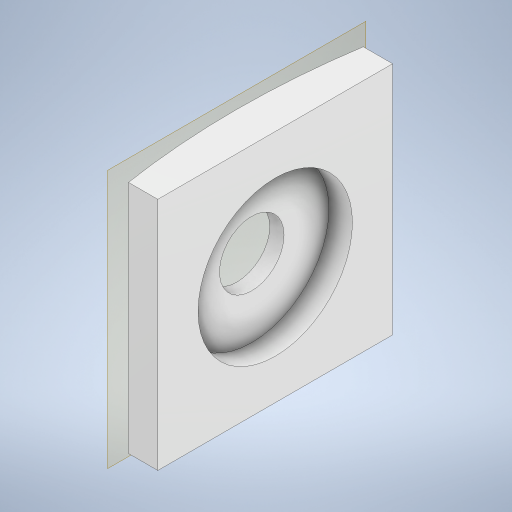
# Autodesk Inventor part: shift_fixed_socket
Saved by Autodesk Inventor 2023 (Build 270158000, 158)
## iProperties
Created: 2023-07-22
Part Number: shift_fixed_socket
Material: Acetal Resin, White
Document SubType Name: Modeling
Designer: 310611102
Density: 1.425 g/cm^3
Appearance: Smooth - White
Mass: 10.3879 g
Surface Area: 43.1103 cm^2
Volume: 7.28974 cm^3
Author: 310611102
Autodesk Inventor part; units mm, degrees
ref_plane "XZ Plane" through (0, 0, 0) normal (0, 1, 0) x (-1, 0, 0)
ref_plane "XY Plane" through (0, 0, 0) normal (0, 0, 1) x (1, 0, 0)
sketch "Sketch1" plane through (0, 0, 0) normal (0, 1, 0) x (-1, 0, 0)
  arc A0 (128.4523, -20) -> (128.4523, 20) centre (0, 0) ccw
  line L0 (128.4523, 20) -> (123.4523, 20)
  line L1 (123.4523, 20) -> (123.4523, -20)
  line L2 (123.4523, -20) -> (128.4523, -20)
  point P0 (123.4523, 0)
  dimension "d0" = 130
  dimension "d1" = 40
  dimension "d2" = 5
  constraints: 6 end point, 2 perpendicular, 2 point on circle, 1 centre point, 1 coincident, 1 horizontal, 1 horizontal alignment, 1 midpoint
  measures "d0" radius of A0
  measures "d1" distance of L0.end L1.end
  measures "d2" distance of L1.end L2.end
extrude "Extrusion1" add sketch "Sketch1" along normal blind 40
sketch "Sketch2" plane through (-123.4523, 0, 20) normal (1, 0, 0) x (0, 0, -1)
  circle A0 centre (20, 20) radius 13.15
  line L0 (0, 0) -> (0, 40) projected
  line L1 (0, 0) -> (40, 0) projected
  point P0 (20, 0)
  point P1 (0, 20)
  point P2 (20, 0)
  dimension "d5" = 26.3
  constraints: 2 midpoint, 1 centre point, 1 horizontal alignment, 1 vertical alignment
  measures "d5" diameter of A0
extrude "Extrusion2" cut sketch "Sketch2" against normal blind 4
sketch "Sketch3" plane through (-127.4523, 20, 0) normal (1, 0, 0) x (0, 0, -1)
  circle A0 centre (0, 0) radius 5.5
  point P0 (0, -20)
  dimension "d8" = 11
  constraints: 1 centre point
  measures "d8" diameter of A0
extrude "Extrusion3" cut sketch "Sketch3" against normal through all
ref_plane "Work Plane1" through (-130, 0, 0) normal (1, 0, 0) x (0, 1, 0)
sketch "Sketch4" plane through (-130, 0, 0) normal (1, 0, 0) x (0, 1, 0)
  circle A0 centre (34.1421, -14.1421) radius 1.5
  circle A1 centre (20, 0) radius 5.5 projected
  circle A2 centre (20, 0) radius 20 construction
  circle A3 centre (34.1421, 14.1421) radius 1.5
  circle A4 centre (5.8579, 14.1421) radius 1.5
  circle A5 centre (5.8579, -14.1421) radius 1.5
  line L0 (20, 0) -> (20, -24.623) construction
  line L1 (20, 0) -> (34.1421, -14.1421) construction
  point P0 (0, 0)
  dimension "d15" = 40
  dimension "d11" = 3
  dimension "d18" = 360
  dimension "d20" = 45
  constraints: 4 centre point, 4 end point, 1 coincident, 1 vertical, 12 other
  measures "d11" diameter of A0
  measures "d20" angle of L0 L1
extrude "Extrusion4" cut sketch "Sketch4" along normal blind 1 contours A0 | A3 | A4 | A5
body "Solid1"
